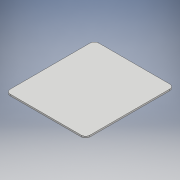
# Autodesk Inventor part: Ventana
Saved by Autodesk Inventor 2017 (Build 210142000, 142)
## iProperties
Part Number: Ventana
Material: Genérico
Document SubType Name: Modeling
Designer: Ghost
Density: 1 g/cm^3
Appearance: Valor por defecto
Author: Ghost
Autodesk Inventor part; units mm, degrees
ref_plane "YZ Plane" through (0, 0, 0) normal (1, 0, 0) x (0, 1, 0)
ref_plane "XZ Plane" through (0, 0, 0) normal (0, 1, 0) x (-1, 0, 0)
ref_plane "XY Plane" through (0, 0, 0) normal (0, 0, 1) x (1, 0, 0)
sketch "Boceto1" plane through (0, 0, 0) normal (0, 0, 1) x (1, 0, 0)
  line L0 (2, 0) -> (35.804, 0)
  line L1 (37.804, 2) -> (37.804, 40)
  line L2 (35.804, 42) -> (2, 42)
  line L3 (0, 40) -> (0, 2)
  arc A0 (2, 42) -> (0, 40) centre (2, 40) ccw
  arc A1 (37.804, 40) -> (35.804, 42) centre (35.804, 40) ccw
  arc A2 (35.804, 0) -> (37.804, 2) centre (35.804, 2) ccw
  arc A3 (0, 2) -> (2, 0) centre (2, 2) ccw
  point P0 (0, 0)
  point P1 (37.804, 0)
  point P2 (0, 42)
  dimension "d2" = 2
  dimension "d7" = 37.804
  dimension "d8" = 42
  constraints: 8 end point, 8 point on circle, 8 tangent, 6 point on line, 4 centre point, 3 equal radius, 2 perpendicular, 1 horizontal, 1 vertical
  measures "d2" radius of A0
  measures "d7" distance between parallel lines of L3 L1
  measures "d8" distance from line of L0 L2.end
extrude "Extrusión1" add sketch "Boceto1" along normal blind 0.75
